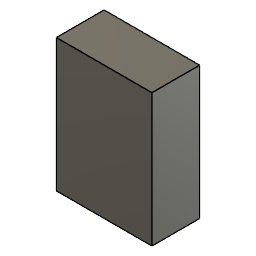
speeduino+mock (Autodesk Fusion 360 design; units mm, degrees)
part number: 2026-02-08-15-26-22-404
Autodesk Fusion 360 part; units mm, degrees
sketch "Sketch1" plane through (0, 0, 0) normal (0, 0, 1) x (1, 0, 0)
  line L0 (-42.3554, 32.3304) -> (27.4946, 32.3304)
  line L1 (27.4946, 32.3304) -> (27.4946, -126.4196)
  line L2 (27.4946, -126.4196) -> (-42.3554, -126.4196)
  line L3 (-42.3554, -126.4196) -> (-42.3554, 32.3304)
  dimension "d1" = 69.85
  dimension "d2" = 158.75
  constraint horizontal L0
  constraint vertical L1
  constraint horizontal L2
  constraint vertical L3
  measures "d1" distance of L0.start L0.end
  measures "d2" distance of L0.start L2.end
extrude "Extrude1" add sketch "Sketch1" along normal blind 57.15
extrude "Extrude2" add 1 faces at (-42.3554, -20.5862, 38.1) along direction (-1, 0, 0) blind 44.45
